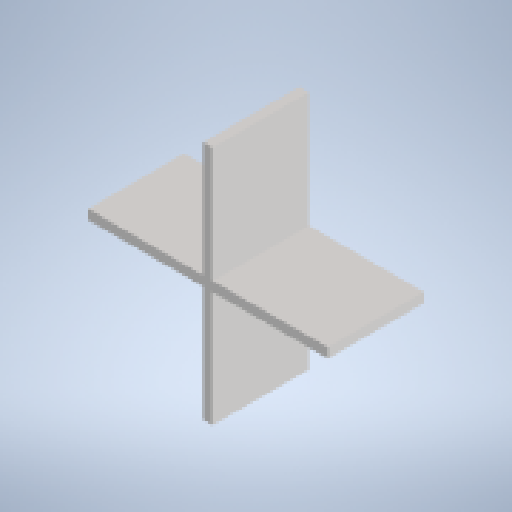
# Autodesk Inventor part: крепление шеи1
Saved by Autodesk Inventor 2023.1 (Build 271208000, 208)
## iProperties
Created: 2024-11-21
Part Number: крепление шеи1
Material: Типовые
Document SubType Name: Modeling
Designer: DELL
Density: 1 g/cm^3
Appearance: По умолчанию
Author: DELL
Autodesk Inventor part; units mm, degrees
ref_plane "YZ Plane" through (0, 0, 0) normal (1, 0, 0) x (0, 1, 0)
ref_plane "XZ Plane" through (0, 0, 0) normal (0, 1, 0) x (-1, 0, 0)
ref_plane "XY Plane" through (0, 0, 0) normal (0, 0, 1) x (1, 0, 0)
sketch "Эскиз1" plane through (0, 0, 0) normal (0, 0, 1) x (1, 0, 0)
  circle A0 centre (0, 0) radius 75 construction
  line L0 (2, -50) -> (-2, -50)
  line L1 (-2, -50) -> (-2, 50)
  line L2 (-2, 50) -> (2, 50)
  line L3 (2, 50) -> (2, -50)
  line L4 (2, -50) -> (-2, 50) construction
  line L5 (-2, -50) -> (2, 50) construction
  line L6 (50, 2) -> (-50, 2)
  line L7 (-50, 2) -> (-50, -2)
  line L8 (-50, -2) -> (50, -2)
  line L9 (50, -2) -> (50, 2)
  line L10 (50, 2) -> (-50, -2) construction
  line L11 (-50, 2) -> (50, -2) construction
  point P0 (-2, 2)
  point P1 (-2, -2)
  point P2 (2, -2)
  point P3 (2, 2)
  dimension "d0" = 150
  dimension "d1" = 4
  dimension "d2" = 100
  dimension "d3" = 100
  dimension "d4" = 4
  constraints: 24 end point, 4 midpoint, 4 parallel, 2 horizontal, 2 perpendicular, 1 centre point, 1 coincident
  measures "d0" diameter of A0
  measures "d1" distance of L1.end L2.end
  measures "d2" distance of L0.end L1.end
  measures "d3" distance of L8.end L7.end
  measures "d4" distance of L7.end L6.end
extrude "Выдавливание1" add sketch "Эскиз1" along normal blind 40
